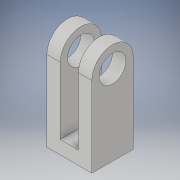
# Autodesk Inventor part: CollecterHolderShort
Saved by Autodesk Inventor 2017 (Build 210142000, 142)
## iProperties
Created: 2017-05-06
Part Number: CollecterHolderShort
Material: Generic
Document SubType Name: Modeling
Designer: User
Density: 1 g/cm^3
Appearance: Default
Author: User
Autodesk Inventor part; units mm, degrees
ref_plane "YZ Plane" through (0, 0, 0) normal (1, 0, 0) x (0, 1, 0)
ref_plane "XZ Plane" through (0, 0, 0) normal (0, 1, 0) x (-1, 0, 0)
ref_plane "XY Plane" through (0, 0, 0) normal (0, 0, 1) x (1, 0, 0)
sketch "Sketch1" plane through (0, 0, 0) normal (1, 0, 0) x (0, 1, 0)
  circle A0 centre (0, 0) radius 6.35
  arc A1 (0, -9.779) -> (0, 9.779) centre (0, 0) ccw
  line L0 (0, 9.779) -> (-38.1, 9.779)
  line L1 (-38.1, 9.779) -> (-38.1, -9.779)
  line L2 (-38.1, -9.779) -> (0, -9.779)
  dimension "d0" = 12.7
  dimension "d1" = 19.558
  dimension "d2" = 38.1
  dimension "d3" = 19.558
  constraints: 6 end point, 2 centre point, 2 coincident, 2 perpendicular, 2 point on circle, 1 horizontal, 1 tangent
  measures "d0" diameter of A0
  measures "d1" diameter of A1
  measures "d2" distance of L0.start L0.end
  measures "d3" distance of L0.end L1.end
extrude "Extrusion1" add sketch "Sketch1" along normal blind 21.336
sketch "Sketch2" plane through (0, -38.1, 9.779) normal (0, 0, 1) x (1, 0, 0)
  line L0 (0, 0) -> (0, 38.1) projected
  line L1 (0, 0) -> (21.336, 0) projected
  line L2 (21.336, 38.1) -> (21.336, 0) projected
  line L3 (0, 38.1) -> (21.336, 38.1) projected
  line L4 (0, 38.1) -> (0, 38.1) projected
  line L5 (0, 38.1) -> (21.336, 38.1) projected
  line L6 (21.336, 38.1) -> (21.336, 38.1) projected
  line L7 (0, 38.1) -> (21.336, 38.1) projected
  line L8 (21.336, 38.1) -> (21.336, 47.879) projected
  line L9 (0, 47.879) -> (21.336, 47.879) projected
  line L10 (6.35, 47.879) -> (6.35, 6.35)
  line L11 (14.986, 47.879) -> (14.986, 6.35)
  line L12 (14.986, 6.35) -> (6.35, 6.35)
  dimension "d6" = 41.529
  dimension "d7" = 6.35
  dimension "d8" = 6.35
  constraints: 6 end point, 2 point on line, 2 vertical, 1 perpendicular
  measures "d6" distance of L10.start L10.end
  measures "d7" distance between parallel lines of L0 L10
  measures "d8" distance between parallel lines of L2 L11
extrude "Extrusion2" cut sketch "Sketch2" against normal blind 21.336 contours L10 L9 L11 L3 | L3 L11 L12 L10
body "Solid1"
